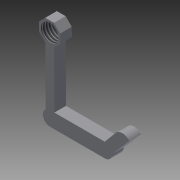
# Autodesk Inventor part: Servo_Arm_Hook_F
Saved by Autodesk Inventor 2015 SP2 (Build 190223200, 223)
## iProperties
Created: 2016-09-13
Part Number: Servo_Arm_Hook_F
Material: Generic
Document SubType Name: Modeling
Designer: jm799
Density: 1 g/cm^3
Appearance: Default
Author: jm799
Autodesk Inventor part; units mm, degrees
ref_plane "YZ Plane" through (0, 0, 0) normal (1, 0, 0) x (0, 1, 0)
ref_plane "XZ Plane" through (0, 0, 0) normal (0, 1, 0) x (-1, 0, 0)
ref_plane "XY Plane" through (0, 0, 0) normal (0, 0, 1) x (1, 0, 0)
ref_plane "Work Plane1" through (0, 7, 0) normal (0, 1, 0) x (1, 0, 0)
sketch "Sketch3" plane through (0, 7, 0) normal (0, 1, 0) x (1, 0, 0)
  line L0 (1.8253, 0.7457) -> (1.818, -0.7634)
  line L1 (1.818, -0.7634) -> (0.7457, -1.8253)
  line L2 (0.7457, -1.8253) -> (-0.7634, -1.818)
  line L3 (-0.7634, -1.818) -> (-1.8253, -0.7457)
  line L4 (-1.8253, -0.7457) -> (-1.818, 0.7634)
  line L5 (-1.818, 0.7634) -> (-0.7457, 1.8253)
  line L6 (-0.7457, 1.8253) -> (0.7634, 1.818)
  line L7 (0.7634, 1.818) -> (1.8253, 0.7457)
  line L8 (-1.8216, 0.0088) -> (1.8216, -0.0088) construction
  line L9 (-0.0088, -1.8216) -> (0.0088, 1.8216) construction
  point P0 (0, 0)
  point P1 (0, 0)
  point P2 (0, 0)
  point P3 (0, 0)
  constraints: 20 end point, 6 midpoint, 2 coincident, 17 other
extrude "Extrusion2" add sketch "Sketch3" along normal blind 2
ref_plane "Work Plane2" through (-0.7457, 7, -1.8253) normal (0.0048553, 0, -0.9999882) x (-0.9999882, 0, -0.0048553)
sketch "Sketch4" plane through (-0.7457, 7, -1.8253) normal (0.0048553, 0, -0.9999882) x (-0.9999882, 0, -0.0048553)
  line L0 (-1.5091, 2) -> (0, 2)
  line L1 (0, 2) -> (0, 0)
  line L2 (0, 0) -> (-1.5091, 0)
  line L3 (-1.5091, 0) -> (-1.5091, 2)
  point P0 (-0.7546, -7)
  constraints: 8 end point, 2 parallel, 1 horizontal, 1 perpendicular
extrude "Extrusion3" add sketch "Sketch4" along normal blind 10
sketch "Sketch5" plane through (0, 9, 0) normal (0, 1, 0) x (1, 0, 0)
  point P0 (0, 0)
sketch "Sketch6" plane through (0, 9, 0) normal (0, 1, 0) x (1, 0, 0)
  point P0 (0, 0)
sketch "Sketch7" plane through (0, 9, 0) normal (0, 1, 0) x (1, 0, 0)
  circle A0 centre (0.062, 12.7642) radius 1.2414
  point P0 (0, 0)
  constraints: 1 centre point
extrude "Extrusion4" add sketch "Sketch7" against normal blind 2
sketch "Sketch8" plane through (0, 9, 0) normal (0, 1, 0) x (1, 0, 0)
  point P0 (0, 0)
sketch "Sketch9" plane through (0, 9, 0) normal (0, 1, 0) x (1, 0, 0)
  point P0 (0, 0)
sketch "Sketch11" plane through (0, 9, 0) normal (0, 1, 0) x (1, 0, 0)
  point P0 (0, 0)
sketch "Sketch12" plane through (0, 9, 0) normal (0, 1, 0) x (1, 0, 0)
  point P0 (0, 0)
ref_plane "Work Plane3" through (0, 9, 0) normal (0, 1, 0) x (1, 0, 0)
sketch "Sketch13" plane through (0, 9, 0) normal (0, 1, 0) x (1, 0, 0)
  line L0 (0.062, 11.5229) -> (9.5019, 11.5229)
  line L1 (0.062, 11.5229) -> (0.062, 14.0056)
  arc A0 (0.8117, 11.7749) -> (-0.6974, 11.7822) centre (0.062, 12.7642) ccw projected
  line L2 (0.062, 14.0056) -> (9.5019, 14.0056)
  line L3 (9.5019, 11.5229) -> (9.5019, 14.0056)
  point P0 (0, 0)
  constraints: 8 end point, 2 horizontal, 2 vertical, 1 point on circle, 1 tangent
extrude "Extrusion6" add sketch "Sketch13" against normal blind 2
ref_plane "Work Plane4" through (0, 9, 0) normal (0, 1, 0) x (1, 0, 0)
sketch "Sketch14" plane through (0, 9, 0) normal (0, 1, 0) x (1, 0, 0)
  line L0 (9.5019, 14.0056) -> (9.5019, 11.5229) projected
  circle A0 centre (9.5019, 12.7642) radius 1.2415
  point P0 (0, 0)
  dimension "d17" = 2.483
  constraints: 1 centre point, 1 midpoint
  measures "d17" diameter of A0
extrude "Extrusion7" add sketch "Sketch14" against normal blind 2
ref_plane "Work Plane5" through (0, 9, 0) normal (0, 1, 0) x (1, 0, 0)
sketch "Sketch15" plane through (0, 9, 0) normal (0, 1, 0) x (1, 0, 0)
  arc A0 (9.4834, 11.5229) -> (9.4834, 14.0056) centre (9.5019, 12.7642) ccw projected
  line L0 (10.7434, 12.7642) -> (13.7224, 9.3009)
  line L1 (9.4834, 11.5229) -> (11.3674, 9.2776)
  line L2 (9.4834, 11.5229) -> (12.4144, 11.5229) construction
  arc A1 (11.3674, 9.2776) -> (13.7224, 9.3009) centre (12.5353, 10.2576) ccw
  point P0 (0, 0)
  dimension "d20" = 50
  constraints: 6 end point, 3 point on circle, 1 centre point, 1 equal length, 1 horizontal, 1 tangent
  measures "d20" angle of L1 L2
extrude "Extrusion8" add sketch "Sketch15" against normal blind 2
sketch "Sketch16" plane through (0, 9, 0) normal (0, 1, 0) x (1, 0, 0)
  point P0 (0, 0)
hole "Hole1" at (0, 9, 0) direction (0, -1, 0) diameter 3 end through all
thread "Thread2" size "M3x0.5" class "6H" standard "ANSI Metric M Profile" full length
body "Solid1"
